Autodesk Inventor part; units mm, degrees
(part 2 of 3)
ref_plane "to_Bolt_1_26_ZX" through (-190.1914, 0, -250) normal (0, 0, -1) x (0, 1, 0)
ref_plane "to_Bolt_1_260_XY" through (-132.7751, 0, 250) normal (0, 1, 0) x (1, 0, 0)
ref_plane "to_Bolt_1_260_YZ" through (-132.7751, 0, 250) normal (1, 0, 0) x (0, 0, -1)
ref_plane "to_Bolt_1_260_ZX" through (-132.7751, 0, 250) normal (0, 0, -1) x (0, 1, 0)
ref_plane "to_Bolt_1_261_XY" through (-130.3828, 0, 250) normal (0, 1, 0) x (1, 0, 0)
ref_plane "to_Bolt_1_261_YZ" through (-130.3828, 0, 250) normal (1, 0, 0) x (0, 0, -1)
ref_plane "to_Bolt_1_261_ZX" through (-130.3828, 0, 250) normal (0, 0, -1) x (0, 1, 0)
ref_plane "to_Bolt_1_262_XY" through (-127.9904, 0, 250) normal (0, 1, 0) x (1, 0, 0)
ref_plane "to_Bolt_1_262_YZ" through (-127.9904, 0, 250) normal (1, 0, 0) x (0, 0, -1)
ref_plane "to_Bolt_1_262_ZX" through (-127.9904, 0, 250) normal (0, 0, -1) x (0, 1, 0)
ref_plane "to_Bolt_1_263_XY" through (-125.5981, 0, 250) normal (0, 1, 0) x (1, 0, 0)
ref_plane "to_Bolt_1_263_YZ" through (-125.5981, 0, 250) normal (1, 0, 0) x (0, 0, -1)
ref_plane "to_Bolt_1_263_ZX" through (-125.5981, 0, 250) normal (0, 0, -1) x (0, 1, 0)
ref_plane "to_Bolt_1_264_XY" through (-123.2057, 0, 250) normal (0, 1, 0) x (1, 0, 0)
ref_plane "to_Bolt_1_264_YZ" through (-123.2057, 0, 250) normal (1, 0, 0) x (0, 0, -1)
ref_plane "to_Bolt_1_264_ZX" through (-123.2057, 0, 250) normal (0, 0, -1) x (0, 1, 0)
ref_plane "to_Bolt_1_265_XY" through (-120.8134, 0, 250) normal (0, 1, 0) x (1, 0, 0)
ref_plane "to_Bolt_1_265_YZ" through (-120.8134, 0, 250) normal (1, 0, 0) x (0, 0, -1)
ref_plane "to_Bolt_1_265_ZX" through (-120.8134, 0, 250) normal (0, 0, -1) x (0, 1, 0)
ref_plane "to_Bolt_1_266_XY" through (-118.4211, 0, 250) normal (0, 1, 0) x (1, 0, 0)
ref_plane "to_Bolt_1_266_YZ" through (-118.4211, 0, 250) normal (1, 0, 0) x (0, 0, -1)
ref_plane "to_Bolt_1_266_ZX" through (-118.4211, 0, 250) normal (0, 0, -1) x (0, 1, 0)
ref_plane "to_Bolt_1_267_XY" through (-116.0287, 0, 250) normal (0, 1, 0) x (1, 0, 0)
ref_plane "to_Bolt_1_267_YZ" through (-116.0287, 0, 250) normal (1, 0, 0) x (0, 0, -1)
ref_plane "to_Bolt_1_267_ZX" through (-116.0287, 0, 250) normal (0, 0, -1) x (0, 1, 0)
ref_plane "to_Bolt_1_268_XY" through (-113.6364, 0, 250) normal (0, 1, 0) x (1, 0, 0)
ref_plane "to_Bolt_1_268_YZ" through (-113.6364, 0, 250) normal (1, 0, 0) x (0, 0, -1)
ref_plane "to_Bolt_1_268_ZX" through (-113.6364, 0, 250) normal (0, 0, -1) x (0, 1, 0)
ref_plane "to_Bolt_1_269_XY" through (-111.244, 0, 250) normal (0, 1, 0) x (1, 0, 0)
ref_plane "to_Bolt_1_269_YZ" through (-111.244, 0, 250) normal (1, 0, 0) x (0, 0, -1)
ref_plane "to_Bolt_1_269_ZX" through (-111.244, 0, 250) normal (0, 0, -1) x (0, 1, 0)
ref_plane "to_Bolt_1_27_XY" through (-187.799, 0, -250) normal (0, 1, 0) x (1, 0, 0)
ref_plane "to_Bolt_1_27_YZ" through (-187.799, 0, -250) normal (1, 0, 0) x (0, 0, -1)
ref_plane "to_Bolt_1_27_ZX" through (-187.799, 0, -250) normal (0, 0, -1) x (0, 1, 0)
ref_plane "to_Bolt_1_270_XY" through (-108.8517, 0, 250) normal (0, 1, 0) x (1, 0, 0)
ref_plane "to_Bolt_1_270_YZ" through (-108.8517, 0, 250) normal (1, 0, 0) x (0, 0, -1)
ref_plane "to_Bolt_1_270_ZX" through (-108.8517, 0, 250) normal (0, 0, -1) x (0, 1, 0)
ref_plane "to_Bolt_1_271_XY" through (-106.4593, 0, 250) normal (0, 1, 0) x (1, 0, 0)
ref_plane "to_Bolt_1_271_YZ" through (-106.4593, 0, 250) normal (1, 0, 0) x (0, 0, -1)
ref_plane "to_Bolt_1_271_ZX" through (-106.4593, 0, 250) normal (0, 0, -1) x (0, 1, 0)
ref_plane "to_Bolt_1_272_XY" through (-104.067, 0, 250) normal (0, 1, 0) x (1, 0, 0)
ref_plane "to_Bolt_1_272_YZ" through (-104.067, 0, 250) normal (1, 0, 0) x (0, 0, -1)
ref_plane "to_Bolt_1_272_ZX" through (-104.067, 0, 250) normal (0, 0, -1) x (0, 1, 0)
ref_plane "to_Bolt_1_273_XY" through (-101.6746, 0, 250) normal (0, 1, 0) x (1, 0, 0)
ref_plane "to_Bolt_1_273_YZ" through (-101.6746, 0, 250) normal (1, 0, 0) x (0, 0, -1)
ref_plane "to_Bolt_1_273_ZX" through (-101.6746, 0, 250) normal (0, 0, -1) x (0, 1, 0)
ref_plane "to_Bolt_1_274_XY" through (-99.2823, 0, 250) normal (0, 1, 0) x (1, 0, 0)
ref_plane "to_Bolt_1_274_YZ" through (-99.2823, 0, 250) normal (1, 0, 0) x (0, 0, -1)
ref_plane "to_Bolt_1_274_ZX" through (-99.2823, 0, 250) normal (0, 0, -1) x (0, 1, 0)
ref_plane "to_Bolt_1_275_XY" through (-96.89, 0, 250) normal (0, 1, 0) x (1, 0, 0)
ref_plane "to_Bolt_1_275_YZ" through (-96.89, 0, 250) normal (1, 0, 0) x (0, 0, -1)
ref_plane "to_Bolt_1_275_ZX" through (-96.89, 0, 250) normal (0, 0, -1) x (0, 1, 0)
ref_plane "to_Bolt_1_276_XY" through (-94.4976, 0, 250) normal (0, 1, 0) x (1, 0, 0)
ref_plane "to_Bolt_1_276_YZ" through (-94.4976, 0, 250) normal (1, 0, 0) x (0, 0, -1)
ref_plane "to_Bolt_1_276_ZX" through (-94.4976, 0, 250) normal (0, 0, -1) x (0, 1, 0)
ref_plane "to_Bolt_1_277_XY" through (-92.1053, 0, 250) normal (0, 1, 0) x (1, 0, 0)
ref_plane "to_Bolt_1_277_YZ" through (-92.1053, 0, 250) normal (1, 0, 0) x (0, 0, -1)
ref_plane "to_Bolt_1_277_ZX" through (-92.1053, 0, 250) normal (0, 0, -1) x (0, 1, 0)
ref_plane "to_Bolt_1_278_XY" through (-89.7129, 0, 250) normal (0, 1, 0) x (1, 0, 0)
ref_plane "to_Bolt_1_278_YZ" through (-89.7129, 0, 250) normal (1, 0, 0) x (0, 0, -1)
ref_plane "to_Bolt_1_278_ZX" through (-89.7129, 0, 250) normal (0, 0, -1) x (0, 1, 0)
ref_plane "to_Bolt_1_279_XY" through (-87.3206, 0, 250) normal (0, 1, 0) x (1, 0, 0)
ref_plane "to_Bolt_1_279_YZ" through (-87.3206, 0, 250) normal (1, 0, 0) x (0, 0, -1)
ref_plane "to_Bolt_1_279_ZX" through (-87.3206, 0, 250) normal (0, 0, -1) x (0, 1, 0)
ref_plane "to_Bolt_1_28_XY" through (-185.4067, 0, -250) normal (0, 1, 0) x (1, 0, 0)
ref_plane "to_Bolt_1_28_YZ" through (-185.4067, 0, -250) normal (1, 0, 0) x (0, 0, -1)
ref_plane "to_Bolt_1_28_ZX" through (-185.4067, 0, -250) normal (0, 0, -1) x (0, 1, 0)
ref_plane "to_Bolt_1_280_XY" through (-84.9282, 0, 250) normal (0, 1, 0) x (1, 0, 0)
ref_plane "to_Bolt_1_280_YZ" through (-84.9282, 0, 250) normal (1, 0, 0) x (0, 0, -1)
ref_plane "to_Bolt_1_280_ZX" through (-84.9282, 0, 250) normal (0, 0, -1) x (0, 1, 0)
ref_plane "to_Bolt_1_281_XY" through (-82.5359, 0, 250) normal (0, 1, 0) x (1, 0, 0)
ref_plane "to_Bolt_1_281_YZ" through (-82.5359, 0, 250) normal (1, 0, 0) x (0, 0, -1)
ref_plane "to_Bolt_1_281_ZX" through (-82.5359, 0, 250) normal (0, 0, -1) x (0, 1, 0)
ref_plane "to_Bolt_1_282_XY" through (-80.1435, 0, 250) normal (0, 1, 0) x (1, 0, 0)
ref_plane "to_Bolt_1_282_YZ" through (-80.1435, 0, 250) normal (1, 0, 0) x (0, 0, -1)
ref_plane "to_Bolt_1_282_ZX" through (-80.1435, 0, 250) normal (0, 0, -1) x (0, 1, 0)
ref_plane "to_Bolt_1_283_XY" through (-77.7512, 0, 250) normal (0, 1, 0) x (1, 0, 0)
ref_plane "to_Bolt_1_283_YZ" through (-77.7512, 0, 250) normal (1, 0, 0) x (0, 0, -1)
ref_plane "to_Bolt_1_283_ZX" through (-77.7512, 0, 250) normal (0, 0, -1) x (0, 1, 0)
ref_plane "to_Bolt_1_284_XY" through (-75.3589, 0, 250) normal (0, 1, 0) x (1, 0, 0)
ref_plane "to_Bolt_1_284_YZ" through (-75.3589, 0, 250) normal (1, 0, 0) x (0, 0, -1)
ref_plane "to_Bolt_1_284_ZX" through (-75.3589, 0, 250) normal (0, 0, -1) x (0, 1, 0)
ref_plane "to_Bolt_1_285_XY" through (-72.9665, 0, 250) normal (0, 1, 0) x (1, 0, 0)
ref_plane "to_Bolt_1_285_YZ" through (-72.9665, 0, 250) normal (1, 0, 0) x (0, 0, -1)
ref_plane "to_Bolt_1_285_ZX" through (-72.9665, 0, 250) normal (0, 0, -1) x (0, 1, 0)
ref_plane "to_Bolt_1_286_XY" through (-70.5742, 0, 250) normal (0, 1, 0) x (1, 0, 0)
ref_plane "to_Bolt_1_286_YZ" through (-70.5742, 0, 250) normal (1, 0, 0) x (0, 0, -1)
ref_plane "to_Bolt_1_286_ZX" through (-70.5742, 0, 250) normal (0, 0, -1) x (0, 1, 0)
ref_plane "to_Bolt_1_287_XY" through (-68.1818, 0, 250) normal (0, 1, 0) x (1, 0, 0)
ref_plane "to_Bolt_1_287_YZ" through (-68.1818, 0, 250) normal (1, 0, 0) x (0, 0, -1)
ref_plane "to_Bolt_1_287_ZX" through (-68.1818, 0, 250) normal (0, 0, -1) x (0, 1, 0)
ref_plane "to_Bolt_1_288_XY" through (-65.7895, 0, 250) normal (0, 1, 0) x (1, 0, 0)
ref_plane "to_Bolt_1_288_YZ" through (-65.7895, 0, 250) normal (1, 0, 0) x (0, 0, -1)
ref_plane "to_Bolt_1_288_ZX" through (-65.7895, 0, 250) normal (0, 0, -1) x (0, 1, 0)
ref_plane "to_Bolt_1_289_XY" through (-63.3971, 0, 250) normal (0, 1, 0) x (1, 0, 0)
ref_plane "to_Bolt_1_289_YZ" through (-63.3971, 0, 250) normal (1, 0, 0) x (0, 0, -1)
ref_plane "to_Bolt_1_289_ZX" through (-63.3971, 0, 250) normal (0, 0, -1) x (0, 1, 0)
ref_plane "to_Bolt_1_29_XY" through (-183.0144, 0, -250) normal (0, 1, 0) x (1, 0, 0)
ref_plane "to_Bolt_1_29_YZ" through (-183.0144, 0, -250) normal (1, 0, 0) x (0, 0, -1)
ref_plane "to_Bolt_1_29_ZX" through (-183.0144, 0, -250) normal (0, 0, -1) x (0, 1, 0)
ref_plane "to_Bolt_1_290_XY" through (-61.0048, 0, 250) normal (0, 1, 0) x (1, 0, 0)
ref_plane "to_Bolt_1_290_YZ" through (-61.0048, 0, 250) normal (1, 0, 0) x (0, 0, -1)
ref_plane "to_Bolt_1_290_ZX" through (-61.0048, 0, 250) normal (0, 0, -1) x (0, 1, 0)
ref_plane "to_Bolt_1_291_XY" through (-58.6124, 0, 250) normal (0, 1, 0) x (1, 0, 0)
ref_plane "to_Bolt_1_291_YZ" through (-58.6124, 0, 250) normal (1, 0, 0) x (0, 0, -1)
ref_plane "to_Bolt_1_291_ZX" through (-58.6124, 0, 250) normal (0, 0, -1) x (0, 1, 0)
ref_plane "to_Bolt_1_292_XY" through (-56.2201, 0, 250) normal (0, 1, 0) x (1, 0, 0)
ref_plane "to_Bolt_1_292_YZ" through (-56.2201, 0, 250) normal (1, 0, 0) x (0, 0, -1)
ref_plane "to_Bolt_1_292_ZX" through (-56.2201, 0, 250) normal (0, 0, -1) x (0, 1, 0)
ref_plane "to_Bolt_1_293_XY" through (-53.8278, 0, 250) normal (0, 1, 0) x (1, 0, 0)
ref_plane "to_Bolt_1_293_YZ" through (-53.8278, 0, 250) normal (1, 0, 0) x (0, 0, -1)
ref_plane "to_Bolt_1_293_ZX" through (-53.8278, 0, 250) normal (0, 0, -1) x (0, 1, 0)
ref_plane "to_Bolt_1_294_XY" through (-51.4354, 0, 250) normal (0, 1, 0) x (1, 0, 0)
ref_plane "to_Bolt_1_294_YZ" through (-51.4354, 0, 250) normal (1, 0, 0) x (0, 0, -1)
ref_plane "to_Bolt_1_294_ZX" through (-51.4354, 0, 250) normal (0, 0, -1) x (0, 1, 0)
ref_plane "to_Bolt_1_295_XY" through (-49.0431, 0, 250) normal (0, 1, 0) x (1, 0, 0)
ref_plane "to_Bolt_1_295_YZ" through (-49.0431, 0, 250) normal (1, 0, 0) x (0, 0, -1)
ref_plane "to_Bolt_1_295_ZX" through (-49.0431, 0, 250) normal (0, 0, -1) x (0, 1, 0)
ref_plane "to_Bolt_1_296_XY" through (-46.6507, 0, 250) normal (0, 1, 0) x (1, 0, 0)
ref_plane "to_Bolt_1_296_YZ" through (-46.6507, 0, 250) normal (1, 0, 0) x (0, 0, -1)
ref_plane "to_Bolt_1_296_ZX" through (-46.6507, 0, 250) normal (0, 0, -1) x (0, 1, 0)
ref_plane "to_Bolt_1_297_XY" through (-44.2584, 0, 250) normal (0, 1, 0) x (1, 0, 0)
ref_plane "to_Bolt_1_297_YZ" through (-44.2584, 0, 250) normal (1, 0, 0) x (0, 0, -1)
ref_plane "to_Bolt_1_297_ZX" through (-44.2584, 0, 250) normal (0, 0, -1) x (0, 1, 0)
ref_plane "to_Bolt_1_298_XY" through (-41.866, 0, 250) normal (0, 1, 0) x (1, 0, 0)
ref_plane "to_Bolt_1_298_YZ" through (-41.866, 0, 250) normal (1, 0, 0) x (0, 0, -1)
ref_plane "to_Bolt_1_298_ZX" through (-41.866, 0, 250) normal (0, 0, -1) x (0, 1, 0)
ref_plane "to_Bolt_1_299_XY" through (-39.4737, 0, 250) normal (0, 1, 0) x (1, 0, 0)
ref_plane "to_Bolt_1_299_YZ" through (-39.4737, 0, 250) normal (1, 0, 0) x (0, 0, -1)
ref_plane "to_Bolt_1_299_ZX" through (-39.4737, 0, 250) normal (0, 0, -1) x (0, 1, 0)
ref_plane "to_Bolt_1_3_XY" through (-245.2153, 0, -250) normal (0, 1, 0) x (1, 0, 0)
ref_plane "to_Bolt_1_3_YZ" through (-245.2153, 0, -250) normal (1, 0, 0) x (0, 0, -1)
ref_plane "to_Bolt_1_3_ZX" through (-245.2153, 0, -250) normal (0, 0, -1) x (0, 1, 0)
ref_plane "to_Bolt_1_30_XY" through (-180.622, 0, -250) normal (0, 1, 0) x (1, 0, 0)
ref_plane "to_Bolt_1_30_YZ" through (-180.622, 0, -250) normal (1, 0, 0) x (0, 0, -1)
ref_plane "to_Bolt_1_30_ZX" through (-180.622, 0, -250) normal (0, 0, -1) x (0, 1, 0)
ref_plane "to_Bolt_1_300_XY" through (-37.0813, 0, 250) normal (0, 1, 0) x (1, 0, 0)
ref_plane "to_Bolt_1_300_YZ" through (-37.0813, 0, 250) normal (1, 0, 0) x (0, 0, -1)
ref_plane "to_Bolt_1_300_ZX" through (-37.0813, 0, 250) normal (0, 0, -1) x (0, 1, 0)
ref_plane "to_Bolt_1_301_XY" through (-34.689, 0, 250) normal (0, 1, 0) x (1, 0, 0)
ref_plane "to_Bolt_1_301_YZ" through (-34.689, 0, 250) normal (1, 0, 0) x (0, 0, -1)
ref_plane "to_Bolt_1_301_ZX" through (-34.689, 0, 250) normal (0, 0, -1) x (0, 1, 0)
ref_plane "to_Bolt_1_302_XY" through (-32.2967, 0, 250) normal (0, 1, 0) x (1, 0, 0)
ref_plane "to_Bolt_1_302_YZ" through (-32.2967, 0, 250) normal (1, 0, 0) x (0, 0, -1)
ref_plane "to_Bolt_1_302_ZX" through (-32.2967, 0, 250) normal (0, 0, -1) x (0, 1, 0)
ref_plane "to_Bolt_1_303_XY" through (-29.9043, 0, 250) normal (0, 1, 0) x (1, 0, 0)
ref_plane "to_Bolt_1_303_YZ" through (-29.9043, 0, 250) normal (1, 0, 0) x (0, 0, -1)
ref_plane "to_Bolt_1_303_ZX" through (-29.9043, 0, 250) normal (0, 0, -1) x (0, 1, 0)
ref_plane "to_Bolt_1_304_XY" through (-27.512, 0, 250) normal (0, 1, 0) x (1, 0, 0)
ref_plane "to_Bolt_1_304_YZ" through (-27.512, 0, 250) normal (1, 0, 0) x (0, 0, -1)
ref_plane "to_Bolt_1_304_ZX" through (-27.512, 0, 250) normal (0, 0, -1) x (0, 1, 0)
ref_plane "to_Bolt_1_305_XY" through (-25.1196, 0, 250) normal (0, 1, 0) x (1, 0, 0)
ref_plane "to_Bolt_1_305_YZ" through (-25.1196, 0, 250) normal (1, 0, 0) x (0, 0, -1)
ref_plane "to_Bolt_1_305_ZX" through (-25.1196, 0, 250) normal (0, 0, -1) x (0, 1, 0)
ref_plane "to_Bolt_1_306_XY" through (-22.7273, 0, 250) normal (0, 1, 0) x (1, 0, 0)
ref_plane "to_Bolt_1_306_YZ" through (-22.7273, 0, 250) normal (1, 0, 0) x (0, 0, -1)
ref_plane "to_Bolt_1_306_ZX" through (-22.7273, 0, 250) normal (0, 0, -1) x (0, 1, 0)
ref_plane "to_Bolt_1_307_XY" through (-20.3349, 0, 250) normal (0, 1, 0) x (1, 0, 0)
ref_plane "to_Bolt_1_307_YZ" through (-20.3349, 0, 250) normal (1, 0, 0) x (0, 0, -1)
ref_plane "to_Bolt_1_307_ZX" through (-20.3349, 0, 250) normal (0, 0, -1) x (0, 1, 0)
ref_plane "to_Bolt_1_308_XY" through (-17.9426, 0, 250) normal (0, 1, 0) x (1, 0, 0)
ref_plane "to_Bolt_1_308_YZ" through (-17.9426, 0, 250) normal (1, 0, 0) x (0, 0, -1)
ref_plane "to_Bolt_1_308_ZX" through (-17.9426, 0, 250) normal (0, 0, -1) x (0, 1, 0)
ref_plane "to_Bolt_1_309_XY" through (-15.5502, 0, 250) normal (0, 1, 0) x (1, 0, 0)
ref_plane "to_Bolt_1_309_YZ" through (-15.5502, 0, 250) normal (1, 0, 0) x (0, 0, -1)
ref_plane "to_Bolt_1_309_ZX" through (-15.5502, 0, 250) normal (0, 0, -1) x (0, 1, 0)
ref_plane "to_Bolt_1_31_XY" through (-178.2297, 0, -250) normal (0, 1, 0) x (1, 0, 0)
ref_plane "to_Bolt_1_31_YZ" through (-178.2297, 0, -250) normal (1, 0, 0) x (0, 0, -1)
ref_plane "to_Bolt_1_31_ZX" through (-178.2297, 0, -250) normal (0, 0, -1) x (0, 1, 0)
ref_plane "to_Bolt_1_310_XY" through (-13.1579, 0, 250) normal (0, 1, 0) x (1, 0, 0)
ref_plane "to_Bolt_1_310_YZ" through (-13.1579, 0, 250) normal (1, 0, 0) x (0, 0, -1)
ref_plane "to_Bolt_1_310_ZX" through (-13.1579, 0, 250) normal (0, 0, -1) x (0, 1, 0)
ref_plane "to_Bolt_1_311_XY" through (-10.7656, 0, 250) normal (0, 1, 0) x (1, 0, 0)
ref_plane "to_Bolt_1_311_YZ" through (-10.7656, 0, 250) normal (1, 0, 0) x (0, 0, -1)
ref_plane "to_Bolt_1_311_ZX" through (-10.7656, 0, 250) normal (0, 0, -1) x (0, 1, 0)
ref_plane "to_Bolt_1_312_XY" through (-8.3732, 0, 250) normal (0, 1, 0) x (1, 0, 0)
ref_plane "to_Bolt_1_312_YZ" through (-8.3732, 0, 250) normal (1, 0, 0) x (0, 0, -1)
ref_plane "to_Bolt_1_312_ZX" through (-8.3732, 0, 250) normal (0, 0, -1) x (0, 1, 0)
ref_plane "to_Bolt_1_313_XY" through (-5.9809, 0, 250) normal (0, 1, 0) x (1, 0, 0)
ref_plane "to_Bolt_1_313_YZ" through (-5.9809, 0, 250) normal (1, 0, 0) x (0, 0, -1)
ref_plane "to_Bolt_1_313_ZX" through (-5.9809, 0, 250) normal (0, 0, -1) x (0, 1, 0)
ref_plane "to_Bolt_1_314_XY" through (-3.5885, 0, 250) normal (0, 1, 0) x (1, 0, 0)
ref_plane "to_Bolt_1_314_YZ" through (-3.5885, 0, 250) normal (1, 0, 0) x (0, 0, -1)
ref_plane "to_Bolt_1_314_ZX" through (-3.5885, 0, 250) normal (0, 0, -1) x (0, 1, 0)
ref_plane "to_Bolt_1_315_XY" through (-1.1962, 0, 250) normal (0, 1, 0) x (1, 0, 0)
ref_plane "to_Bolt_1_315_YZ" through (-1.1962, 0, 250) normal (1, 0, 0) x (0, 0, -1)
ref_plane "to_Bolt_1_315_ZX" through (-1.1962, 0, 250) normal (0, 0, -1) x (0, 1, 0)
ref_plane "to_Bolt_1_316_XY" through (1.1962, 0, 250) normal (0, 1, 0) x (1, 0, 0)
ref_plane "to_Bolt_1_316_YZ" through (1.1962, 0, 250) normal (1, 0, 0) x (0, 0, -1)
ref_plane "to_Bolt_1_316_ZX" through (1.1962, 0, 250) normal (0, 0, -1) x (0, 1, 0)
ref_plane "to_Bolt_1_317_XY" through (3.5885, 0, 250) normal (0, 1, 0) x (1, 0, 0)
ref_plane "to_Bolt_1_317_YZ" through (3.5885, 0, 250) normal (1, 0, 0) x (0, 0, -1)
ref_plane "to_Bolt_1_317_ZX" through (3.5885, 0, 250) normal (0, 0, -1) x (0, 1, 0)
ref_plane "to_Bolt_1_318_XY" through (5.9809, 0, 250) normal (0, 1, 0) x (1, 0, 0)
ref_plane "to_Bolt_1_318_YZ" through (5.9809, 0, 250) normal (1, 0, 0) x (0, 0, -1)
ref_plane "to_Bolt_1_318_ZX" through (5.9809, 0, 250) normal (0, 0, -1) x (0, 1, 0)
ref_plane "to_Bolt_1_319_XY" through (8.3732, 0, 250) normal (0, 1, 0) x (1, 0, 0)
ref_plane "to_Bolt_1_319_YZ" through (8.3732, 0, 250) normal (1, 0, 0) x (0, 0, -1)
ref_plane "to_Bolt_1_319_ZX" through (8.3732, 0, 250) normal (0, 0, -1) x (0, 1, 0)
ref_plane "to_Bolt_1_32_XY" through (-175.8373, 0, -250) normal (0, 1, 0) x (1, 0, 0)
ref_plane "to_Bolt_1_32_YZ" through (-175.8373, 0, -250) normal (1, 0, 0) x (0, 0, -1)
ref_plane "to_Bolt_1_32_ZX" through (-175.8373, 0, -250) normal (0, 0, -1) x (0, 1, 0)
ref_plane "to_Bolt_1_320_XY" through (10.7656, 0, 250) normal (0, 1, 0) x (1, 0, 0)
ref_plane "to_Bolt_1_320_YZ" through (10.7656, 0, 250) normal (1, 0, 0) x (0, 0, -1)
ref_plane "to_Bolt_1_320_ZX" through (10.7656, 0, 250) normal (0, 0, -1) x (0, 1, 0)
ref_plane "to_Bolt_1_321_XY" through (13.1579, 0, 250) normal (0, 1, 0) x (1, 0, 0)
ref_plane "to_Bolt_1_321_YZ" through (13.1579, 0, 250) normal (1, 0, 0) x (0, 0, -1)
ref_plane "to_Bolt_1_321_ZX" through (13.1579, 0, 250) normal (0, 0, -1) x (0, 1, 0)
ref_plane "to_Bolt_1_322_XY" through (15.5502, 0, 250) normal (0, 1, 0) x (1, 0, 0)
ref_plane "to_Bolt_1_322_YZ" through (15.5502, 0, 250) normal (1, 0, 0) x (0, 0, -1)
ref_plane "to_Bolt_1_322_ZX" through (15.5502, 0, 250) normal (0, 0, -1) x (0, 1, 0)
ref_plane "to_Bolt_1_323_XY" through (17.9426, 0, 250) normal (0, 1, 0) x (1, 0, 0)
ref_plane "to_Bolt_1_323_YZ" through (17.9426, 0, 250) normal (1, 0, 0) x (0, 0, -1)
ref_plane "to_Bolt_1_323_ZX" through (17.9426, 0, 250) normal (0, 0, -1) x (0, 1, 0)
ref_plane "to_Bolt_1_324_XY" through (20.3349, 0, 250) normal (0, 1, 0) x (1, 0, 0)
ref_plane "to_Bolt_1_324_YZ" through (20.3349, 0, 250) normal (1, 0, 0) x (0, 0, -1)
ref_plane "to_Bolt_1_324_ZX" through (20.3349, 0, 250) normal (0, 0, -1) x (0, 1, 0)
ref_plane "to_Bolt_1_325_XY" through (22.7273, 0, 250) normal (0, 1, 0) x (1, 0, 0)
ref_plane "to_Bolt_1_325_YZ" through (22.7273, 0, 250) normal (1, 0, 0) x (0, 0, -1)
ref_plane "to_Bolt_1_325_ZX" through (22.7273, 0, 250) normal (0, 0, -1) x (0, 1, 0)
ref_plane "to_Bolt_1_326_XY" through (25.1196, 0, 250) normal (0, 1, 0) x (1, 0, 0)
ref_plane "to_Bolt_1_326_YZ" through (25.1196, 0, 250) normal (1, 0, 0) x (0, 0, -1)
ref_plane "to_Bolt_1_326_ZX" through (25.1196, 0, 250) normal (0, 0, -1) x (0, 1, 0)
ref_plane "to_Bolt_1_327_XY" through (27.512, 0, 250) normal (0, 1, 0) x (1, 0, 0)
ref_plane "to_Bolt_1_327_YZ" through (27.512, 0, 250) normal (1, 0, 0) x (0, 0, -1)
ref_plane "to_Bolt_1_327_ZX" through (27.512, 0, 250) normal (0, 0, -1) x (0, 1, 0)
ref_plane "to_Bolt_1_328_XY" through (29.9043, 0, 250) normal (0, 1, 0) x (1, 0, 0)
ref_plane "to_Bolt_1_328_YZ" through (29.9043, 0, 250) normal (1, 0, 0) x (0, 0, -1)
ref_plane "to_Bolt_1_328_ZX" through (29.9043, 0, 250) normal (0, 0, -1) x (0, 1, 0)
ref_plane "to_Bolt_1_329_XY" through (32.2967, 0, 250) normal (0, 1, 0) x (1, 0, 0)
ref_plane "to_Bolt_1_329_YZ" through (32.2967, 0, 250) normal (1, 0, 0) x (0, 0, -1)
ref_plane "to_Bolt_1_329_ZX" through (32.2967, 0, 250) normal (0, 0, -1) x (0, 1, 0)
ref_plane "to_Bolt_1_33_XY" through (-173.445, 0, -250) normal (0, 1, 0) x (1, 0, 0)
ref_plane "to_Bolt_1_33_YZ" through (-173.445, 0, -250) normal (1, 0, 0) x (0, 0, -1)
ref_plane "to_Bolt_1_33_ZX" through (-173.445, 0, -250) normal (0, 0, -1) x (0, 1, 0)
ref_plane "to_Bolt_1_330_XY" through (34.689, 0, 250) normal (0, 1, 0) x (1, 0, 0)
ref_plane "to_Bolt_1_330_YZ" through (34.689, 0, 250) normal (1, 0, 0) x (0, 0, -1)
ref_plane "to_Bolt_1_330_ZX" through (34.689, 0, 250) normal (0, 0, -1) x (0, 1, 0)
ref_plane "to_Bolt_1_331_XY" through (37.0813, 0, 250) normal (0, 1, 0) x (1, 0, 0)
ref_plane "to_Bolt_1_331_YZ" through (37.0813, 0, 250) normal (1, 0, 0) x (0, 0, -1)
ref_plane "to_Bolt_1_331_ZX" through (37.0813, 0, 250) normal (0, 0, -1) x (0, 1, 0)
ref_plane "to_Bolt_1_332_XY" through (39.4737, 0, 250) normal (0, 1, 0) x (1, 0, 0)
ref_plane "to_Bolt_1_332_YZ" through (39.4737, 0, 250) normal (1, 0, 0) x (0, 0, -1)
ref_plane "to_Bolt_1_332_ZX" through (39.4737, 0, 250) normal (0, 0, -1) x (0, 1, 0)
ref_plane "to_Bolt_1_333_XY" through (41.866, 0, 250) normal (0, 1, 0) x (1, 0, 0)
ref_plane "to_Bolt_1_333_YZ" through (41.866, 0, 250) normal (1, 0, 0) x (0, 0, -1)
ref_plane "to_Bolt_1_333_ZX" through (41.866, 0, 250) normal (0, 0, -1) x (0, 1, 0)
ref_plane "to_Bolt_1_334_XY" through (44.2584, 0, 250) normal (0, 1, 0) x (1, 0, 0)
ref_plane "to_Bolt_1_334_YZ" through (44.2584, 0, 250) normal (1, 0, 0) x (0, 0, -1)
ref_plane "to_Bolt_1_334_ZX" through (44.2584, 0, 250) normal (0, 0, -1) x (0, 1, 0)
ref_plane "to_Bolt_1_335_XY" through (46.6507, 0, 250) normal (0, 1, 0) x (1, 0, 0)
ref_plane "to_Bolt_1_335_YZ" through (46.6507, 0, 250) normal (1, 0, 0) x (0, 0, -1)
ref_plane "to_Bolt_1_335_ZX" through (46.6507, 0, 250) normal (0, 0, -1) x (0, 1, 0)
ref_plane "to_Bolt_1_336_XY" through (49.0431, 0, 250) normal (0, 1, 0) x (1, 0, 0)
ref_plane "to_Bolt_1_336_YZ" through (49.0431, 0, 250) normal (1, 0, 0) x (0, 0, -1)
ref_plane "to_Bolt_1_336_ZX" through (49.0431, 0, 250) normal (0, 0, -1) x (0, 1, 0)
ref_plane "to_Bolt_1_337_XY" through (51.4354, 0, 250) normal (0, 1, 0) x (1, 0, 0)
ref_plane "to_Bolt_1_337_YZ" through (51.4354, 0, 250) normal (1, 0, 0) x (0, 0, -1)
ref_plane "to_Bolt_1_337_ZX" through (51.4354, 0, 250) normal (0, 0, -1) x (0, 1, 0)
ref_plane "to_Bolt_1_338_XY" through (53.8278, 0, 250) normal (0, 1, 0) x (1, 0, 0)
ref_plane "to_Bolt_1_338_YZ" through (53.8278, 0, 250) normal (1, 0, 0) x (0, 0, -1)
ref_plane "to_Bolt_1_338_ZX" through (53.8278, 0, 250) normal (0, 0, -1) x (0, 1, 0)
ref_plane "to_Bolt_1_339_XY" through (56.2201, 0, 250) normal (0, 1, 0) x (1, 0, 0)
ref_plane "to_Bolt_1_339_YZ" through (56.2201, 0, 250) normal (1, 0, 0) x (0, 0, -1)
ref_plane "to_Bolt_1_339_ZX" through (56.2201, 0, 250) normal (0, 0, -1) x (0, 1, 0)
ref_plane "to_Bolt_1_34_XY" through (-171.0526, 0, -250) normal (0, 1, 0) x (1, 0, 0)
ref_plane "to_Bolt_1_34_YZ" through (-171.0526, 0, -250) normal (1, 0, 0) x (0, 0, -1)
ref_plane "to_Bolt_1_34_ZX" through (-171.0526, 0, -250) normal (0, 0, -1) x (0, 1, 0)
ref_plane "to_Bolt_1_340_XY" through (58.6124, 0, 250) normal (0, 1, 0) x (1, 0, 0)
ref_plane "to_Bolt_1_340_YZ" through (58.6124, 0, 250) normal (1, 0, 0) x (0, 0, -1)
ref_plane "to_Bolt_1_340_ZX" through (58.6124, 0, 250) normal (0, 0, -1) x (0, 1, 0)
ref_plane "to_Bolt_1_341_XY" through (61.0048, 0, 250) normal (0, 1, 0) x (1, 0, 0)
ref_plane "to_Bolt_1_341_YZ" through (61.0048, 0, 250) normal (1, 0, 0) x (0, 0, -1)
ref_plane "to_Bolt_1_341_ZX" through (61.0048, 0, 250) normal (0, 0, -1) x (0, 1, 0)
ref_plane "to_Bolt_1_342_XY" through (63.3971, 0, 250) normal (0, 1, 0) x (1, 0, 0)
ref_plane "to_Bolt_1_342_YZ" through (63.3971, 0, 250) normal (1, 0, 0) x (0, 0, -1)
ref_plane "to_Bolt_1_342_ZX" through (63.3971, 0, 250) normal (0, 0, -1) x (0, 1, 0)
ref_plane "to_Bolt_1_343_XY" through (65.7895, 0, 250) normal (0, 1, 0) x (1, 0, 0)
ref_plane "to_Bolt_1_343_YZ" through (65.7895, 0, 250) normal (1, 0, 0) x (0, 0, -1)
ref_plane "to_Bolt_1_343_ZX" through (65.7895, 0, 250) normal (0, 0, -1) x (0, 1, 0)
ref_plane "to_Bolt_1_344_XY" through (68.1818, 0, 250) normal (0, 1, 0) x (1, 0, 0)
ref_plane "to_Bolt_1_344_YZ" through (68.1818, 0, 250) normal (1, 0, 0) x (0, 0, -1)
ref_plane "to_Bolt_1_344_ZX" through (68.1818, 0, 250) normal (0, 0, -1) x (0, 1, 0)
ref_plane "to_Bolt_1_345_XY" through (70.5742, 0, 250) normal (0, 1, 0) x (1, 0, 0)
ref_plane "to_Bolt_1_345_YZ" through (70.5742, 0, 250) normal (1, 0, 0) x (0, 0, -1)
ref_plane "to_Bolt_1_345_ZX" through (70.5742, 0, 250) normal (0, 0, -1) x (0, 1, 0)
ref_plane "to_Bolt_1_346_XY" through (72.9665, 0, 250) normal (0, 1, 0) x (1, 0, 0)
ref_plane "to_Bolt_1_346_YZ" through (72.9665, 0, 250) normal (1, 0, 0) x (0, 0, -1)
ref_plane "to_Bolt_1_346_ZX" through (72.9665, 0, 250) normal (0, 0, -1) x (0, 1, 0)
ref_plane "to_Bolt_1_347_XY" through (75.3589, 0, 250) normal (0, 1, 0) x (1, 0, 0)
ref_plane "to_Bolt_1_347_YZ" through (75.3589, 0, 250) normal (1, 0, 0) x (0, 0, -1)
ref_plane "to_Bolt_1_347_ZX" through (75.3589, 0, 250) normal (0, 0, -1) x (0, 1, 0)
ref_plane "to_Bolt_1_348_XY" through (77.7512, 0, 250) normal (0, 1, 0) x (1, 0, 0)
ref_plane "to_Bolt_1_348_YZ" through (77.7512, 0, 250) normal (1, 0, 0) x (0, 0, -1)
ref_plane "to_Bolt_1_348_ZX" through (77.7512, 0, 250) normal (0, 0, -1) x (0, 1, 0)
ref_plane "to_Bolt_1_349_XY" through (80.1435, 0, 250) normal (0, 1, 0) x (1, 0, 0)
ref_plane "to_Bolt_1_349_YZ" through (80.1435, 0, 250) normal (1, 0, 0) x (0, 0, -1)
ref_plane "to_Bolt_1_349_ZX" through (80.1435, 0, 250) normal (0, 0, -1) x (0, 1, 0)
ref_plane "to_Bolt_1_35_XY" through (-168.6603, 0, -250) normal (0, 1, 0) x (1, 0, 0)
ref_plane "to_Bolt_1_35_YZ" through (-168.6603, 0, -250) normal (1, 0, 0) x (0, 0, -1)
ref_plane "to_Bolt_1_35_ZX" through (-168.6603, 0, -250) normal (0, 0, -1) x (0, 1, 0)
ref_plane "to_Bolt_1_350_XY" through (82.5359, 0, 250) normal (0, 1, 0) x (1, 0, 0)
ref_plane "to_Bolt_1_350_YZ" through (82.5359, 0, 250) normal (1, 0, 0) x (0, 0, -1)
ref_plane "to_Bolt_1_350_ZX" through (82.5359, 0, 250) normal (0, 0, -1) x (0, 1, 0)
ref_plane "to_Bolt_1_351_XY" through (84.9282, 0, 250) normal (0, 1, 0) x (1, 0, 0)
ref_plane "to_Bolt_1_351_YZ" through (84.9282, 0, 250) normal (1, 0, 0) x (0, 0, -1)
ref_plane "to_Bolt_1_351_ZX" through (84.9282, 0, 250) normal (0, 0, -1) x (0, 1, 0)
ref_plane "to_Bolt_1_352_XY" through (87.3206, 0, 250) normal (0, 1, 0) x (1, 0, 0)
ref_plane "to_Bolt_1_352_YZ" through (87.3206, 0, 250) normal (1, 0, 0) x (0, 0, -1)
ref_plane "to_Bolt_1_352_ZX" through (87.3206, 0, 250) normal (0, 0, -1) x (0, 1, 0)
ref_plane "to_Bolt_1_353_XY" through (89.7129, 0, 250) normal (0, 1, 0) x (1, 0, 0)
ref_plane "to_Bolt_1_353_YZ" through (89.7129, 0, 250) normal (1, 0, 0) x (0, 0, -1)
ref_plane "to_Bolt_1_353_ZX" through (89.7129, 0, 250) normal (0, 0, -1) x (0, 1, 0)
ref_plane "to_Bolt_1_354_XY" through (92.1053, 0, 250) normal (0, 1, 0) x (1, 0, 0)
ref_plane "to_Bolt_1_354_YZ" through (92.1053, 0, 250) normal (1, 0, 0) x (0, 0, -1)
ref_plane "to_Bolt_1_354_ZX" through (92.1053, 0, 250) normal (0, 0, -1) x (0, 1, 0)
ref_plane "to_Bolt_1_355_XY" through (94.4976, 0, 250) normal (0, 1, 0) x (1, 0, 0)
ref_plane "to_Bolt_1_355_YZ" through (94.4976, 0, 250) normal (1, 0, 0) x (0, 0, -1)
ref_plane "to_Bolt_1_355_ZX" through (94.4976, 0, 250) normal (0, 0, -1) x (0, 1, 0)
ref_plane "to_Bolt_1_356_XY" through (96.89, 0, 250) normal (0, 1, 0) x (1, 0, 0)
ref_plane "to_Bolt_1_356_YZ" through (96.89, 0, 250) normal (1, 0, 0) x (0, 0, -1)
ref_plane "to_Bolt_1_356_ZX" through (96.89, 0, 250) normal (0, 0, -1) x (0, 1, 0)
ref_plane "to_Bolt_1_357_XY" through (99.2823, 0, 250) normal (0, 1, 0) x (1, 0, 0)
ref_plane "to_Bolt_1_357_YZ" through (99.2823, 0, 250) normal (1, 0, 0) x (0, 0, -1)
ref_plane "to_Bolt_1_357_ZX" through (99.2823, 0, 250) normal (0, 0, -1) x (0, 1, 0)
ref_plane "to_Bolt_1_358_XY" through (101.6746, 0, 250) normal (0, 1, 0) x (1, 0, 0)
ref_plane "to_Bolt_1_358_YZ" through (101.6746, 0, 250) normal (1, 0, 0) x (0, 0, -1)
ref_plane "to_Bolt_1_358_ZX" through (101.6746, 0, 250) normal (0, 0, -1) x (0, 1, 0)
ref_plane "to_Bolt_1_359_XY" through (104.067, 0, 250) normal (0, 1, 0) x (1, 0, 0)
ref_plane "to_Bolt_1_359_YZ" through (104.067, 0, 250) normal (1, 0, 0) x (0, 0, -1)
ref_plane "to_Bolt_1_359_ZX" through (104.067, 0, 250) normal (0, 0, -1) x (0, 1, 0)
ref_plane "to_Bolt_1_36_XY" through (-166.2679, 0, -250) normal (0, 1, 0) x (1, 0, 0)
ref_plane "to_Bolt_1_36_YZ" through (-166.2679, 0, -250) normal (1, 0, 0) x (0, 0, -1)
ref_plane "to_Bolt_1_36_ZX" through (-166.2679, 0, -250) normal (0, 0, -1) x (0, 1, 0)
ref_plane "to_Bolt_1_360_XY" through (106.4593, 0, 250) normal (0, 1, 0) x (1, 0, 0)
ref_plane "to_Bolt_1_360_YZ" through (106.4593, 0, 250) normal (1, 0, 0) x (0, 0, -1)
ref_plane "to_Bolt_1_360_ZX" through (106.4593, 0, 250) normal (0, 0, -1) x (0, 1, 0)
ref_plane "to_Bolt_1_361_XY" through (108.8517, 0, 250) normal (0, 1, 0) x (1, 0, 0)
ref_plane "to_Bolt_1_361_YZ" through (108.8517, 0, 250) normal (1, 0, 0) x (0, 0, -1)
ref_plane "to_Bolt_1_361_ZX" through (108.8517, 0, 250) normal (0, 0, -1) x (0, 1, 0)
ref_plane "to_Bolt_1_362_XY" through (111.244, 0, 250) normal (0, 1, 0) x (1, 0, 0)
ref_plane "to_Bolt_1_362_YZ" through (111.244, 0, 250) normal (1, 0, 0) x (0, 0, -1)
ref_plane "to_Bolt_1_362_ZX" through (111.244, 0, 250) normal (0, 0, -1) x (0, 1, 0)
ref_plane "to_Bolt_1_363_XY" through (113.6364, 0, 250) normal (0, 1, 0) x (1, 0, 0)
ref_plane "to_Bolt_1_363_YZ" through (113.6364, 0, 250) normal (1, 0, 0) x (0, 0, -1)
ref_plane "to_Bolt_1_363_ZX" through (113.6364, 0, 250) normal (0, 0, -1) x (0, 1, 0)
ref_plane "to_Bolt_1_364_XY" through (116.0287, 0, 250) normal (0, 1, 0) x (1, 0, 0)
ref_plane "to_Bolt_1_364_YZ" through (116.0287, 0, 250) normal (1, 0, 0) x (0, 0, -1)
ref_plane "to_Bolt_1_364_ZX" through (116.0287, 0, 250) normal (0, 0, -1) x (0, 1, 0)
ref_plane "to_Bolt_1_365_XY" through (118.4211, 0, 250) normal (0, 1, 0) x (1, 0, 0)
ref_plane "to_Bolt_1_365_YZ" through (118.4211, 0, 250) normal (1, 0, 0) x (0, 0, -1)
ref_plane "to_Bolt_1_365_ZX" through (118.4211, 0, 250) normal (0, 0, -1) x (0, 1, 0)
ref_plane "to_Bolt_1_366_XY" through (120.8134, 0, 250) normal (0, 1, 0) x (1, 0, 0)
ref_plane "to_Bolt_1_366_YZ" through (120.8134, 0, 250) normal (1, 0, 0) x (0, 0, -1)
ref_plane "to_Bolt_1_366_ZX" through (120.8134, 0, 250) normal (0, 0, -1) x (0, 1, 0)
ref_plane "to_Bolt_1_367_XY" through (123.2057, 0, 250) normal (0, 1, 0) x (1, 0, 0)
ref_plane "to_Bolt_1_367_YZ" through (123.2057, 0, 250) normal (1, 0, 0) x (0, 0, -1)
ref_plane "to_Bolt_1_367_ZX" through (123.2057, 0, 250) normal (0, 0, -1) x (0, 1, 0)
ref_plane "to_Bolt_1_368_XY" through (125.5981, 0, 250) normal (0, 1, 0) x (1, 0, 0)
ref_plane "to_Bolt_1_368_YZ" through (125.5981, 0, 250) normal (1, 0, 0) x (0, 0, -1)
ref_plane "to_Bolt_1_368_ZX" through (125.5981, 0, 250) normal (0, 0, -1) x (0, 1, 0)
ref_plane "to_Bolt_1_369_XY" through (127.9904, 0, 250) normal (0, 1, 0) x (1, 0, 0)
ref_plane "to_Bolt_1_369_YZ" through (127.9904, 0, 250) normal (1, 0, 0) x (0, 0, -1)
ref_plane "to_Bolt_1_369_ZX" through (127.9904, 0, 250) normal (0, 0, -1) x (0, 1, 0)
ref_plane "to_Bolt_1_37_XY" through (-163.8756, 0, -250) normal (0, 1, 0) x (1, 0, 0)
ref_plane "to_Bolt_1_37_YZ" through (-163.8756, 0, -250) normal (1, 0, 0) x (0, 0, -1)
ref_plane "to_Bolt_1_37_ZX" through (-163.8756, 0, -250) normal (0, 0, -1) x (0, 1, 0)
ref_plane "to_Bolt_1_370_XY" through (130.3828, 0, 250) normal (0, 1, 0) x (1, 0, 0)
ref_plane "to_Bolt_1_370_YZ" through (130.3828, 0, 250) normal (1, 0, 0) x (0, 0, -1)
ref_plane "to_Bolt_1_370_ZX" through (130.3828, 0, 250) normal (0, 0, -1) x (0, 1, 0)
ref_plane "to_Bolt_1_371_XY" through (132.7751, 0, 250) normal (0, 1, 0) x (1, 0, 0)
ref_plane "to_Bolt_1_371_YZ" through (132.7751, 0, 250) normal (1, 0, 0) x (0, 0, -1)
ref_plane "to_Bolt_1_371_ZX" through (132.7751, 0, 250) normal (0, 0, -1) x (0, 1, 0)
ref_plane "to_Bolt_1_372_XY" through (135.1675, 0, 250) normal (0, 1, 0) x (1, 0, 0)
ref_plane "to_Bolt_1_372_YZ" through (135.1675, 0, 250) normal (1, 0, 0) x (0, 0, -1)
ref_plane "to_Bolt_1_372_ZX" through (135.1675, 0, 250) normal (0, 0, -1) x (0, 1, 0)
ref_plane "to_Bolt_1_373_XY" through (137.5598, 0, 250) normal (0, 1, 0) x (1, 0, 0)
ref_plane "to_Bolt_1_373_YZ" through (137.5598, 0, 250) normal (1, 0, 0) x (0, 0, -1)
ref_plane "to_Bolt_1_373_ZX" through (137.5598, 0, 250) normal (0, 0, -1) x (0, 1, 0)
ref_plane "to_Bolt_1_374_XY" through (139.9522, 0, 250) normal (0, 1, 0) x (1, 0, 0)
ref_plane "to_Bolt_1_374_YZ" through (139.9522, 0, 250) normal (1, 0, 0) x (0, 0, -1)
ref_plane "to_Bolt_1_374_ZX" through (139.9522, 0, 250) normal (0, 0, -1) x (0, 1, 0)
ref_plane "to_Bolt_1_375_XY" through (142.3445, 0, 250) normal (0, 1, 0) x (1, 0, 0)
ref_plane "to_Bolt_1_375_YZ" through (142.3445, 0, 250) normal (1, 0, 0) x (0, 0, -1)
ref_plane "to_Bolt_1_375_ZX" through (142.3445, 0, 250) normal (0, 0, -1) x (0, 1, 0)
ref_plane "to_Bolt_1_376_XY" through (144.7368, 0, 250) normal (0, 1, 0) x (1, 0, 0)
ref_plane "to_Bolt_1_376_YZ" through (144.7368, 0, 250) normal (1, 0, 0) x (0, 0, -1)
ref_plane "to_Bolt_1_376_ZX" through (144.7368, 0, 250) normal (0, 0, -1) x (0, 1, 0)
ref_plane "to_Bolt_1_377_XY" through (147.1292, 0, 250) normal (0, 1, 0) x (1, 0, 0)
ref_plane "to_Bolt_1_377_YZ" through (147.1292, 0, 250) normal (1, 0, 0) x (0, 0, -1)
ref_plane "to_Bolt_1_377_ZX" through (147.1292, 0, 250) normal (0, 0, -1) x (0, 1, 0)
ref_plane "to_Bolt_1_378_XY" through (149.5215, 0, 250) normal (0, 1, 0) x (1, 0, 0)
ref_plane "to_Bolt_1_378_YZ" through (149.5215, 0, 250) normal (1, 0, 0) x (0, 0, -1)
ref_plane "to_Bolt_1_378_ZX" through (149.5215, 0, 250) normal (0, 0, -1) x (0, 1, 0)
ref_plane "to_Bolt_1_379_XY" through (151.9139, 0, 250) normal (0, 1, 0) x (1, 0, 0)
ref_plane "to_Bolt_1_379_YZ" through (151.9139, 0, 250) normal (1, 0, 0) x (0, 0, -1)
ref_plane "to_Bolt_1_379_ZX" through (151.9139, 0, 250) normal (0, 0, -1) x (0, 1, 0)
ref_plane "to_Bolt_1_38_XY" through (-161.4833, 0, -250) normal (0, 1, 0) x (1, 0, 0)
ref_plane "to_Bolt_1_38_YZ" through (-161.4833, 0, -250) normal (1, 0, 0) x (0, 0, -1)
ref_plane "to_Bolt_1_38_ZX" through (-161.4833, 0, -250) normal (0, 0, -1) x (0, 1, 0)
ref_plane "to_Bolt_1_380_XY" through (154.3062, 0, 250) normal (0, 1, 0) x (1, 0, 0)
ref_plane "to_Bolt_1_380_YZ" through (154.3062, 0, 250) normal (1, 0, 0) x (0, 0, -1)
ref_plane "to_Bolt_1_380_ZX" through (154.3062, 0, 250) normal (0, 0, -1) x (0, 1, 0)
ref_plane "to_Bolt_1_381_XY" through (156.6986, 0, 250) normal (0, 1, 0) x (1, 0, 0)
ref_plane "to_Bolt_1_381_YZ" through (156.6986, 0, 250) normal (1, 0, 0) x (0, 0, -1)
ref_plane "to_Bolt_1_381_ZX" through (156.6986, 0, 250) normal (0, 0, -1) x (0, 1, 0)
ref_plane "to_Bolt_1_382_XY" through (159.0909, 0, 250) normal (0, 1, 0) x (1, 0, 0)
ref_plane "to_Bolt_1_382_YZ" through (159.0909, 0, 250) normal (1, 0, 0) x (0, 0, -1)
ref_plane "to_Bolt_1_382_ZX" through (159.0909, 0, 250) normal (0, 0, -1) x (0, 1, 0)
ref_plane "to_Bolt_1_383_XY" through (161.4833, 0, 250) normal (0, 1, 0) x (1, 0, 0)
ref_plane "to_Bolt_1_383_YZ" through (161.4833, 0, 250) normal (1, 0, 0) x (0, 0, -1)
ref_plane "to_Bolt_1_383_ZX" through (161.4833, 0, 250) normal (0, 0, -1) x (0, 1, 0)
ref_plane "to_Bolt_1_384_XY" through (163.8756, 0, 250) normal (0, 1, 0) x (1, 0, 0)
ref_plane "to_Bolt_1_384_YZ" through (163.8756, 0, 250) normal (1, 0, 0) x (0, 0, -1)
ref_plane "to_Bolt_1_384_ZX" through (163.8756, 0, 250) normal (0, 0, -1) x (0, 1, 0)
ref_plane "to_Bolt_1_385_XY" through (166.2679, 0, 250) normal (0, 1, 0) x (1, 0, 0)
ref_plane "to_Bolt_1_385_YZ" through (166.2679, 0, 250) normal (1, 0, 0) x (0, 0, -1)
ref_plane "to_Bolt_1_385_ZX" through (166.2679, 0, 250) normal (0, 0, -1) x (0, 1, 0)
ref_plane "to_Bolt_1_386_XY" through (168.6603, 0, 250) normal (0, 1, 0) x (1, 0, 0)
ref_plane "to_Bolt_1_386_YZ" through (168.6603, 0, 250) normal (1, 0, 0) x (0, 0, -1)
ref_plane "to_Bolt_1_386_ZX" through (168.6603, 0, 250) normal (0, 0, -1) x (0, 1, 0)
ref_plane "to_Bolt_1_387_XY" through (171.0526, 0, 250) normal (0, 1, 0) x (1, 0, 0)
ref_plane "to_Bolt_1_387_YZ" through (171.0526, 0, 250) normal (1, 0, 0) x (0, 0, -1)
ref_plane "to_Bolt_1_387_ZX" through (171.0526, 0, 250) normal (0, 0, -1) x (0, 1, 0)
ref_plane "to_Bolt_1_388_XY" through (173.445, 0, 250) normal (0, 1, 0) x (1, 0, 0)
ref_plane "to_Bolt_1_388_YZ" through (173.445, 0, 250) normal (1, 0, 0) x (0, 0, -1)
ref_plane "to_Bolt_1_388_ZX" through (173.445, 0, 250) normal (0, 0, -1) x (0, 1, 0)
ref_plane "to_Bolt_1_389_XY" through (175.8373, 0, 250) normal (0, 1, 0) x (1, 0, 0)
ref_plane "to_Bolt_1_389_YZ" through (175.8373, 0, 250) normal (1, 0, 0) x (0, 0, -1)
ref_plane "to_Bolt_1_389_ZX" through (175.8373, 0, 250) normal (0, 0, -1) x (0, 1, 0)
ref_plane "to_Bolt_1_39_XY" through (-159.0909, 0, -250) normal (0, 1, 0) x (1, 0, 0)
ref_plane "to_Bolt_1_39_YZ" through (-159.0909, 0, -250) normal (1, 0, 0) x (0, 0, -1)
ref_plane "to_Bolt_1_39_ZX" through (-159.0909, 0, -250) normal (0, 0, -1) x (0, 1, 0)
ref_plane "to_Bolt_1_390_XY" through (178.2297, 0, 250) normal (0, 1, 0) x (1, 0, 0)
ref_plane "to_Bolt_1_390_YZ" through (178.2297, 0, 250) normal (1, 0, 0) x (0, 0, -1)
ref_plane "to_Bolt_1_390_ZX" through (178.2297, 0, 250) normal (0, 0, -1) x (0, 1, 0)
ref_plane "to_Bolt_1_391_XY" through (180.622, 0, 250) normal (0, 1, 0) x (1, 0, 0)
ref_plane "to_Bolt_1_391_YZ" through (180.622, 0, 250) normal (1, 0, 0) x (0, 0, -1)
ref_plane "to_Bolt_1_391_ZX" through (180.622, 0, 250) normal (0, 0, -1) x (0, 1, 0)
ref_plane "to_Bolt_1_392_XY" through (183.0144, 0, 250) normal (0, 1, 0) x (1, 0, 0)
ref_plane "to_Bolt_1_392_YZ" through (183.0144, 0, 250) normal (1, 0, 0) x (0, 0, -1)
ref_plane "to_Bolt_1_392_ZX" through (183.0144, 0, 250) normal (0, 0, -1) x (0, 1, 0)
ref_plane "to_Bolt_1_393_XY" through (185.4067, 0, 250) normal (0, 1, 0) x (1, 0, 0)
ref_plane "to_Bolt_1_393_YZ" through (185.4067, 0, 250) normal (1, 0, 0) x (0, 0, -1)
ref_plane "to_Bolt_1_393_ZX" through (185.4067, 0, 250) normal (0, 0, -1) x (0, 1, 0)
ref_plane "to_Bolt_1_394_XY" through (187.799, 0, 250) normal (0, 1, 0) x (1, 0, 0)
ref_plane "to_Bolt_1_394_YZ" through (187.799, 0, 250) normal (1, 0, 0) x (0, 0, -1)
ref_plane "to_Bolt_1_394_ZX" through (187.799, 0, 250) normal (0, 0, -1) x (0, 1, 0)
ref_plane "to_Bolt_1_395_XY" through (190.1914, 0, 250) normal (0, 1, 0) x (1, 0, 0)
ref_plane "to_Bolt_1_395_YZ" through (190.1914, 0, 250) normal (1, 0, 0) x (0, 0, -1)
ref_plane "to_Bolt_1_395_ZX" through (190.1914, 0, 250) normal (0, 0, -1) x (0, 1, 0)
ref_plane "to_Bolt_1_396_XY" through (192.5837, 0, 250) normal (0, 1, 0) x (1, 0, 0)
ref_plane "to_Bolt_1_396_YZ" through (192.5837, 0, 250) normal (1, 0, 0) x (0, 0, -1)
ref_plane "to_Bolt_1_396_ZX" through (192.5837, 0, 250) normal (0, 0, -1) x (0, 1, 0)
ref_plane "to_Bolt_1_397_XY" through (194.9761, 0, 250) normal (0, 1, 0) x (1, 0, 0)
ref_plane "to_Bolt_1_397_YZ" through (194.9761, 0, 250) normal (1, 0, 0) x (0, 0, -1)
ref_plane "to_Bolt_1_397_ZX" through (194.9761, 0, 250) normal (0, 0, -1) x (0, 1, 0)
ref_plane "to_Bolt_1_398_XY" through (197.3684, 0, 250) normal (0, 1, 0) x (1, 0, 0)
ref_plane "to_Bolt_1_398_YZ" through (197.3684, 0, 250) normal (1, 0, 0) x (0, 0, -1)
ref_plane "to_Bolt_1_398_ZX" through (197.3684, 0, 250) normal (0, 0, -1) x (0, 1, 0)
ref_plane "to_Bolt_1_399_XY" through (199.7608, 0, 250) normal (0, 1, 0) x (1, 0, 0)
ref_plane "to_Bolt_1_399_YZ" through (199.7608, 0, 250) normal (1, 0, 0) x (0, 0, -1)
ref_plane "to_Bolt_1_399_ZX" through (199.7608, 0, 250) normal (0, 0, -1) x (0, 1, 0)
ref_plane "to_Bolt_1_4_XY" through (-248.823, 0, -250) normal (0, 1, 0) x (1, 0, 0)
ref_plane "to_Bolt_1_4_YZ" through (-248.823, 0, -250) normal (1, 0, 0) x (0, 0, -1)
ref_plane "to_Bolt_1_4_ZX" through (-248.823, 0, -250) normal (0, 0, -1) x (0, 1, 0)
ref_plane "to_Bolt_1_40_XY" through (-156.6986, 0, -250) normal (0, 1, 0) x (1, 0, 0)
ref_plane "to_Bolt_1_40_YZ" through (-156.6986, 0, -250) normal (1, 0, 0) x (0, 0, -1)
ref_plane "to_Bolt_1_40_ZX" through (-156.6986, 0, -250) normal (0, 0, -1) x (0, 1, 0)
ref_plane "to_Bolt_1_400_XY" through (202.1531, 0, 250) normal (0, 1, 0) x (1, 0, 0)
ref_plane "to_Bolt_1_400_YZ" through (202.1531, 0, 250) normal (1, 0, 0) x (0, 0, -1)
ref_plane "to_Bolt_1_400_ZX" through (202.1531, 0, 250) normal (0, 0, -1) x (0, 1, 0)
ref_plane "to_Bolt_1_401_XY" through (204.5455, 0, 250) normal (0, 1, 0) x (1, 0, 0)
ref_plane "to_Bolt_1_401_YZ" through (204.5455, 0, 250) normal (1, 0, 0) x (0, 0, -1)
ref_plane "to_Bolt_1_401_ZX" through (204.5455, 0, 250) normal (0, 0, -1) x (0, 1, 0)
ref_plane "to_Bolt_1_402_XY" through (206.9378, 0, 250) normal (0, 1, 0) x (1, 0, 0)
ref_plane "to_Bolt_1_402_YZ" through (206.9378, 0, 250) normal (1, 0, 0) x (0, 0, -1)
ref_plane "to_Bolt_1_402_ZX" through (206.9378, 0, 250) normal (0, 0, -1) x (0, 1, 0)
ref_plane "to_Bolt_1_403_XY" through (209.3301, 0, 250) normal (0, 1, 0) x (1, 0, 0)
ref_plane "to_Bolt_1_403_YZ" through (209.3301, 0, 250) normal (1, 0, 0) x (0, 0, -1)
ref_plane "to_Bolt_1_403_ZX" through (209.3301, 0, 250) normal (0, 0, -1) x (0, 1, 0)
ref_plane "to_Bolt_1_404_XY" through (211.7225, 0, 250) normal (0, 1, 0) x (1, 0, 0)
ref_plane "to_Bolt_1_404_YZ" through (211.7225, 0, 250) normal (1, 0, 0) x (0, 0, -1)
ref_plane "to_Bolt_1_404_ZX" through (211.7225, 0, 250) normal (0, 0, -1) x (0, 1, 0)
ref_plane "to_Bolt_1_405_XY" through (214.1148, 0, 250) normal (0, 1, 0) x (1, 0, 0)
ref_plane "to_Bolt_1_405_YZ" through (214.1148, 0, 250) normal (1, 0, 0) x (0, 0, -1)
ref_plane "to_Bolt_1_405_ZX" through (214.1148, 0, 250) normal (0, 0, -1) x (0, 1, 0)
ref_plane "to_Bolt_1_406_XY" through (216.5072, 0, 250) normal (0, 1, 0) x (1, 0, 0)
ref_plane "to_Bolt_1_406_YZ" through (216.5072, 0, 250) normal (1, 0, 0) x (0, 0, -1)
ref_plane "to_Bolt_1_406_ZX" through (216.5072, 0, 250) normal (0, 0, -1) x (0, 1, 0)
ref_plane "to_Bolt_1_407_XY" through (218.8995, 0, 250) normal (0, 1, 0) x (1, 0, 0)
ref_plane "to_Bolt_1_407_YZ" through (218.8995, 0, 250) normal (1, 0, 0) x (0, 0, -1)
ref_plane "to_Bolt_1_407_ZX" through (218.8995, 0, 250) normal (0, 0, -1) x (0, 1, 0)
ref_plane "to_Bolt_1_408_XY" through (221.2919, 0, 250) normal (0, 1, 0) x (1, 0, 0)
ref_plane "to_Bolt_1_408_YZ" through (221.2919, 0, 250) normal (1, 0, 0) x (0, 0, -1)
ref_plane "to_Bolt_1_408_ZX" through (221.2919, 0, 250) normal (0, 0, -1) x (0, 1, 0)
ref_plane "to_Bolt_1_409_XY" through (223.6842, 0, 250) normal (0, 1, 0) x (1, 0, 0)
ref_plane "to_Bolt_1_409_YZ" through (223.6842, 0, 250) normal (1, 0, 0) x (0, 0, -1)
ref_plane "to_Bolt_1_409_ZX" through (223.6842, 0, 250) normal (0, 0, -1) x (0, 1, 0)
ref_plane "to_Bolt_1_41_XY" through (-154.3062, 0, -250) normal (0, 1, 0) x (1, 0, 0)
ref_plane "to_Bolt_1_41_YZ" through (-154.3062, 0, -250) normal (1, 0, 0) x (0, 0, -1)
ref_plane "to_Bolt_1_41_ZX" through (-154.3062, 0, -250) normal (0, 0, -1) x (0, 1, 0)
ref_plane "to_Bolt_1_410_XY" through (226.0766, 0, 250) normal (0, 1, 0) x (1, 0, 0)
ref_plane "to_Bolt_1_410_YZ" through (226.0766, 0, 250) normal (1, 0, 0) x (0, 0, -1)
ref_plane "to_Bolt_1_410_ZX" through (226.0766, 0, 250) normal (0, 0, -1) x (0, 1, 0)
ref_plane "to_Bolt_1_411_XY" through (228.4689, 0, 250) normal (0, 1, 0) x (1, 0, 0)
ref_plane "to_Bolt_1_411_YZ" through (228.4689, 0, 250) normal (1, 0, 0) x (0, 0, -1)
ref_plane "to_Bolt_1_411_ZX" through (228.4689, 0, 250) normal (0, 0, -1) x (0, 1, 0)
ref_plane "to_Bolt_1_412_XY" through (230.8612, 0, 250) normal (0, 1, 0) x (1, 0, 0)
ref_plane "to_Bolt_1_412_YZ" through (230.8612, 0, 250) normal (1, 0, 0) x (0, 0, -1)
ref_plane "to_Bolt_1_412_ZX" through (230.8612, 0, 250) normal (0, 0, -1) x (0, 1, 0)
ref_plane "to_Bolt_1_413_XY" through (233.2536, 0, 250) normal (0, 1, 0) x (1, 0, 0)
ref_plane "to_Bolt_1_413_YZ" through (233.2536, 0, 250) normal (1, 0, 0) x (0, 0, -1)
ref_plane "to_Bolt_1_413_ZX" through (233.2536, 0, 250) normal (0, 0, -1) x (0, 1, 0)
ref_plane "to_Bolt_1_414_XY" through (235.6459, 0, 250) normal (0, 1, 0) x (1, 0, 0)
ref_plane "to_Bolt_1_414_YZ" through (235.6459, 0, 250) normal (1, 0, 0) x (0, 0, -1)
ref_plane "to_Bolt_1_414_ZX" through (235.6459, 0, 250) normal (0, 0, -1) x (0, 1, 0)
ref_plane "to_Bolt_1_415_XY" through (238.0383, 0, 250) normal (0, 1, 0) x (1, 0, 0)
ref_plane "to_Bolt_1_415_YZ" through (238.0383, 0, 250) normal (1, 0, 0) x (0, 0, -1)
ref_plane "to_Bolt_1_415_ZX" through (238.0383, 0, 250) normal (0, 0, -1) x (0, 1, 0)
ref_plane "to_Bolt_1_416_XY" through (240.4306, 0, 250) normal (0, 1, 0) x (1, 0, 0)
ref_plane "to_Bolt_1_416_YZ" through (240.4306, 0, 250) normal (1, 0, 0) x (0, 0, -1)
ref_plane "to_Bolt_1_416_ZX" through (240.4306, 0, 250) normal (0, 0, -1) x (0, 1, 0)
ref_plane "to_Bolt_1_417_XY" through (242.823, 0, 250) normal (0, 1, 0) x (1, 0, 0)
ref_plane "to_Bolt_1_417_YZ" through (242.823, 0, 250) normal (1, 0, 0) x (0, 0, -1)
ref_plane "to_Bolt_1_417_ZX" through (242.823, 0, 250) normal (0, 0, -1) x (0, 1, 0)
ref_plane "to_Bolt_1_418_XY" through (245.2153, 0, 250) normal (0, 1, 0) x (1, 0, 0)
ref_plane "to_Bolt_1_418_YZ" through (245.2153, 0, 250) normal (1, 0, 0) x (0, 0, -1)
ref_plane "to_Bolt_1_418_ZX" through (245.2153, 0, 250) normal (0, 0, -1) x (0, 1, 0)
ref_plane "to_Bolt_1_419_XY" through (247.6077, 0, 250) normal (0, 1, 0) x (1, 0, 0)
ref_plane "to_Bolt_1_419_YZ" through (247.6077, 0, 250) normal (1, 0, 0) x (0, 0, -1)
ref_plane "to_Bolt_1_419_ZX" through (247.6077, 0, 250) normal (0, 0, -1) x (0, 1, 0)
ref_plane "to_Bolt_1_42_XY" through (-151.9139, 0, -250) normal (0, 1, 0) x (1, 0, 0)
ref_plane "to_Bolt_1_42_YZ" through (-151.9139, 0, -250) normal (1, 0, 0) x (0, 0, -1)
ref_plane "to_Bolt_1_42_ZX" through (-151.9139, 0, -250) normal (0, 0, -1) x (0, 1, 0)
ref_plane "to_Bolt_1_420_XY" through (250, 0, 250) normal (0, 1, 0) x (1, 0, 0)
ref_plane "to_Bolt_1_420_YZ" through (250, 0, 250) normal (1, 0, 0) x (0, 0, -1)
ref_plane "to_Bolt_1_420_ZX" through (250, 0, 250) normal (0, 0, -1) x (0, 1, 0)
ref_plane "to_Bolt_1_43_XY" through (-149.5215, 0, -250) normal (0, 1, 0) x (1, 0, 0)
ref_plane "to_Bolt_1_43_YZ" through (-149.5215, 0, -250) normal (1, 0, 0) x (0, 0, -1)
ref_plane "to_Bolt_1_43_ZX" through (-149.5215, 0, -250) normal (0, 0, -1) x (0, 1, 0)
ref_plane "to_Bolt_1_44_XY" through (-147.1292, 0, -250) normal (0, 1, 0) x (1, 0, 0)
ref_plane "to_Bolt_1_44_YZ" through (-147.1292, 0, -250) normal (1, 0, 0) x (0, 0, -1)
ref_plane "to_Bolt_1_44_ZX" through (-147.1292, 0, -250) normal (0, 0, -1) x (0, 1, 0)
ref_plane "to_Bolt_1_45_XY" through (-144.7368, 0, -250) normal (0, 1, 0) x (1, 0, 0)
ref_plane "to_Bolt_1_45_YZ" through (-144.7368, 0, -250) normal (1, 0, 0) x (0, 0, -1)
ref_plane "to_Bolt_1_45_ZX" through (-144.7368, 0, -250) normal (0, 0, -1) x (0, 1, 0)
ref_plane "to_Bolt_1_46_XY" through (-142.3445, 0, -250) normal (0, 1, 0) x (1, 0, 0)
ref_plane "to_Bolt_1_46_YZ" through (-142.3445, 0, -250) normal (1, 0, 0) x (0, 0, -1)
ref_plane "to_Bolt_1_46_ZX" through (-142.3445, 0, -250) normal (0, 0, -1) x (0, 1, 0)
ref_plane "to_Bolt_1_47_XY" through (-139.9522, 0, -250) normal (0, 1, 0) x (1, 0, 0)
ref_plane "to_Bolt_1_47_YZ" through (-139.9522, 0, -250) normal (1, 0, 0) x (0, 0, -1)
ref_plane "to_Bolt_1_47_ZX" through (-139.9522, 0, -250) normal (0, 0, -1) x (0, 1, 0)
ref_plane "to_Bolt_1_48_XY" through (-137.5598, 0, -250) normal (0, 1, 0) x (1, 0, 0)
ref_plane "to_Bolt_1_48_YZ" through (-137.5598, 0, -250) normal (1, 0, 0) x (0, 0, -1)
ref_plane "to_Bolt_1_48_ZX" through (-137.5598, 0, -250) normal (0, 0, -1) x (0, 1, 0)
ref_plane "to_Bolt_1_49_XY" through (-135.1675, 0, -250) normal (0, 1, 0) x (1, 0, 0)
ref_plane "to_Bolt_1_49_YZ" through (-135.1675, 0, -250) normal (1, 0, 0) x (0, 0, -1)
ref_plane "to_Bolt_1_49_ZX" through (-135.1675, 0, -250) normal (0, 0, -1) x (0, 1, 0)
ref_plane "to_Bolt_1_5_XY" through (-234.4306, 0, -250) normal (0, 1, 0) x (1, 0, 0)
ref_plane "to_Bolt_1_5_YZ" through (-234.4306, 0, -250) normal (1, 0, 0) x (0, 0, -1)
ref_plane "to_Bolt_1_5_ZX" through (-234.4306, 0, -250) normal (0, 0, -1) x (0, 1, 0)
ref_plane "to_Bolt_1_50_XY" through (-132.7751, 0, -250) normal (0, 1, 0) x (1, 0, 0)
ref_plane "to_Bolt_1_50_YZ" through (-132.7751, 0, -250) normal (1, 0, 0) x (0, 0, -1)
ref_plane "to_Bolt_1_50_ZX" through (-132.7751, 0, -250) normal (0, 0, -1) x (0, 1, 0)
ref_plane "to_Bolt_1_51_XY" through (-130.3828, 0, -250) normal (0, 1, 0) x (1, 0, 0)
ref_plane "to_Bolt_1_51_YZ" through (-130.3828, 0, -250) normal (1, 0, 0) x (0, 0, -1)
ref_plane "to_Bolt_1_51_ZX" through (-130.3828, 0, -250) normal (0, 0, -1) x (0, 1, 0)
ref_plane "to_Bolt_1_52_XY" through (-127.9904, 0, -250) normal (0, 1, 0) x (1, 0, 0)
ref_plane "to_Bolt_1_52_YZ" through (-127.9904, 0, -250) normal (1, 0, 0) x (0, 0, -1)
ref_plane "to_Bolt_1_52_ZX" through (-127.9904, 0, -250) normal (0, 0, -1) x (0, 1, 0)
ref_plane "to_Bolt_1_53_XY" through (-125.5981, 0, -250) normal (0, 1, 0) x (1, 0, 0)
ref_plane "to_Bolt_1_53_YZ" through (-125.5981, 0, -250) normal (1, 0, 0) x (0, 0, -1)
ref_plane "to_Bolt_1_53_ZX" through (-125.5981, 0, -250) normal (0, 0, -1) x (0, 1, 0)
ref_plane "to_Bolt_1_54_XY" through (-123.2057, 0, -250) normal (0, 1, 0) x (1, 0, 0)
ref_plane "to_Bolt_1_54_YZ" through (-123.2057, 0, -250) normal (1, 0, 0) x (0, 0, -1)
ref_plane "to_Bolt_1_54_ZX" through (-123.2057, 0, -250) normal (0, 0, -1) x (0, 1, 0)
ref_plane "to_Bolt_1_55_XY" through (-120.8134, 0, -250) normal (0, 1, 0) x (1, 0, 0)
ref_plane "to_Bolt_1_55_YZ" through (-120.8134, 0, -250) normal (1, 0, 0) x (0, 0, -1)
ref_plane "to_Bolt_1_55_ZX" through (-120.8134, 0, -250) normal (0, 0, -1) x (0, 1, 0)
ref_plane "to_Bolt_1_56_XY" through (-118.4211, 0, -250) normal (0, 1, 0) x (1, 0, 0)
ref_plane "to_Bolt_1_56_YZ" through (-118.4211, 0, -250) normal (1, 0, 0) x (0, 0, -1)